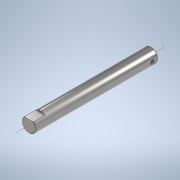
# Autodesk Inventor part: crankshaft
Saved by Autodesk Inventor 2021.1 (Build 251245000, 245)
## iProperties
Created: 2020-08-31
Part Number: crankshaft
Material: Stainless Steel
Document SubType Name: Sheet Metal
Designer: Vamshi
Mass: 1548.82 g
Surface Area: 276.87 cm^2
Volume: 193.602 cm^3
Density: 8 g/cm^3
Sheet Metal Rule: Default
Appearance: Semi-Polished
Author: Vamshi
Autodesk Inventor part; units mm, degrees
ref_plane "YZ Plane" through (0, 0, 0) normal (1, 0, 0) x (0, 1, 0)
ref_plane "XZ Plane" through (0, 0, 0) normal (0, 1, 0) x (-1, 0, 0)
ref_plane "XY Plane" through (0, 0, 0) normal (0, 0, 1) x (1, 0, 0)
sketch "Sketch1" plane through (0, 0, 0) normal (0, 0, 1) x (1, 0, 0)
  circle A0 centre (0, 0) radius 15.24
  dimension "d0" = 30.48
  constraints: 1 centre point, 1 coincident
  measures "d0" diameter of A0
extrude "Extrusion1" add sketch "Sketch1" along normal mid plane 269.24
sketch "Sketch2" plane through (0, 0, 0) normal (1, 0, 0) x (0, 1, 0)
  line L0 (15.24, -134.62) -> (-15.24, -134.62) projected
  line L1 (-15.24, -134.62) -> (-15.24, 134.62) projected
  line L2 (-15.24, 134.62) -> (15.24, 134.62) projected
  line L3 (15.24, 134.62) -> (15.24, -134.62) projected
  line L4 (-15.24, -134.62) -> (15.24, -134.62) projected
  line L5 (15.24, 134.62) -> (-15.24, 134.62) projected
  circle A0 centre (0, -121.92) radius 3.81
  line L6 (19.558, 134.62) -> (11.43, 134.62)
  line L7 (11.43, 134.62) -> (11.43, 109.22)
  line L8 (11.43, 109.22) -> (19.558, 109.22)
  line L9 (19.558, 109.22) -> (19.558, 134.62)
  line L10 (0, -188.468) -> (0, 188.468) projected
  point P0 (0, 0)
  dimension "d3" = 7.62
  dimension "d4" = 12.7
  dimension "d5" = 8.128
  dimension "d6" = 25.4
  dimension "d7" = 11.43
  constraints: 8 end point, 2 parallel, 1 centre point, 1 horizontal, 1 perpendicular, 1 point on line
  measures "d3" diameter of A0
  measures "d4" distance from line of L0 A0.centre
  measures "d5" distance of L8.end L7.end
  measures "d6" distance of L7.end L6.end
  measures "d7" distance between parallel lines of L10 L7
extrude "Extrusion2" cut sketch "Sketch2" against normal through all both and the other way through all contours L8 L7 L2 L3 | L3 L6 L9 L8 | L10 A0 | A0 L10
chamfer "Chamfer1" distance 1.27 angle 45 3 edges at (13.8903, 6.2703, 134.62) (-6.2703, -13.8903, 134.62) (-15.24, 0, -134.62) measured on face at (-13.538, 6.9987, 44.8733)
equation "\"BendRadius\" = Thickness"
equation "\"BendReliefWidth\" = Thickness"
equation "\"BendReliefDepth\" = 0.5 * Thickness"
equation "\"CornerReliefSize\" = 4 * Thickness"
equation "\"MinimumRemnant\" = 2 * Thickness"
equation "\"TransitionRadius\" = BendRadius"
equation "\"JacobiRadiusSize\" = BendRadius"
equation "\"GapSize\" = Thickness"
equation "\"Thickness\" = 3.048"
body "Solid1"
